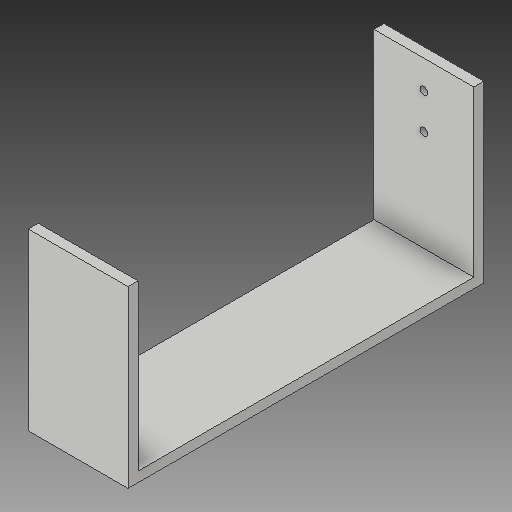
# Autodesk Inventor part: Leg Servo Holder
Saved by Autodesk Inventor 2018 (Build 220112000, 112)
## iProperties
Created: 2018-04-22
Part Number: Leg Servo Holder
Material: Generic
Document SubType Name: Modeling
Designer: HP
Density: 1 g/cm^3
Appearance: Default
Mass: 5.48341 g
Surface Area: 61.3131 cm^2
Volume: 5.48341 cm^3
Author: HP
Autodesk Inventor part; units mm, degrees
ref_plane "YZ Plane" through (0, 0, 0) normal (1, 0, 0) x (0, 1, 0)
ref_plane "XZ Plane" through (0, 0, 0) normal (0, 1, 0) x (-1, 0, 0)
ref_plane "XY Plane" through (0, 0, 0) normal (0, 0, 1) x (1, 0, 0)
sketch "Sketch1" plane through (0, 0, 0) normal (0, 1, 0) x (-1, 0, 0)
  line L0 (0, 0) -> (-20, 0)
  line L1 (-20, 0) -> (-20, -67.262)
  line L2 (-20, -67.262) -> (0, -67.262)
  line L3 (0, -67.262) -> (0, 0)
  dimension "d0" = 20
  dimension "d1" = 67.262
  constraints: 8 end point, 2 parallel, 1 horizontal, 1 perpendicular
  measures "d0" distance of L2.end L1.end
  measures "d1" distance of L1.end L0.end
extrude "Extrusion1" add sketch "Sketch1" along normal blind 2
sketch "Sketch2" plane through (0, 0, 0) normal (0, 0, 1) x (1, 0, 0)
  line L0 (0, 0) -> (20, 0)
  line L1 (20, 0) -> (20, 35)
  line L2 (20, 35) -> (0, 35)
  line L3 (0, 35) -> (0, 0)
  dimension "d4" = 20
  dimension "d5" = 35
  constraints: 8 end point, 2 parallel, 1 horizontal, 1 perpendicular
  measures "d4" distance of L2.end L1.end
  measures "d5" distance of L1.end L0.end
extrude "Extrusion2" add sketch "Sketch2" along normal blind 2
sketch "Sketch4" plane through (20, 0, -67.262) normal (0, 0, -1) x (-1, 0, 0)
  line L0 (0, 35) -> (20, 35) projected
  line L1 (0, 35) -> (20, 35)
  line L2 (20, 35) -> (20, 0)
  line L3 (20, 0) -> (0, 0)
  line L4 (0, 0) -> (0, 35)
  constraints: 8 end point, 2 parallel, 1 horizontal, 1 perpendicular
extrude "Extrusion3" add sketch "Sketch4" along normal blind 2
sketch "Sketch5" plane through (20, 0, -69.262) normal (0, 0, -1) x (-1, 0, 0)
  circle A0 centre (10, 29.36) radius 0.75
  line L0 (20, 35) -> (0, 35) projected
  line L1 (0, 35) -> (0, 0) projected
  point P0 (20, 0)
  dimension "d10" = 1.5
  dimension "d11" = 5.64
  dimension "d12" = 10
  constraints: 1 centre point
  measures "d10" diameter of A0
  measures "d11" distance from line of L0 A0.centre
  measures "d12" distance from line of L1 A0.centre
extrude "Extrusion4" cut sketch "Sketch5" against normal blind 2
sketch "Sketch6" plane through (20, 0, -69.262) normal (0, 0, -1) x (-1, 0, 0)
  circle A0 centre (10, 22.26) radius 0.75
  line L0 (0, 35) -> (0, 0) projected
  circle A1 centre (10, 29.36) radius 0.75 projected
  point P0 (20, 0)
  dimension "d15" = 1.5
  dimension "d16" = 10
  dimension "d17" = 7.1
  constraints: 1 centre point
  measures "d15" diameter of A0
  measures "d16" distance from line of L0 A0.centre
  measures "d17" distance of A1.centre A0.centre
extrude "Extrusion5" cut sketch "Sketch6" against normal blind 2 contours A0
body "Solid1"
